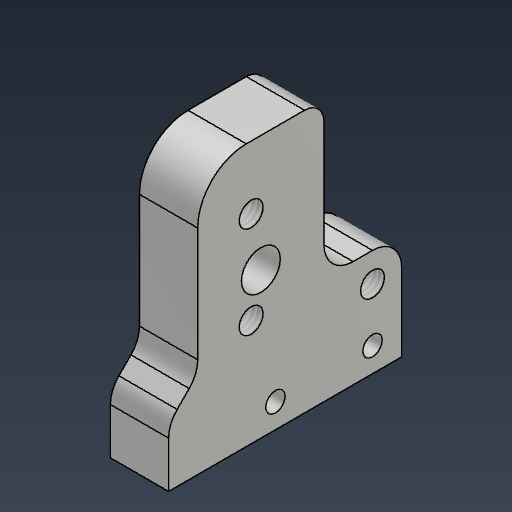
# Autodesk Inventor part: Dribbler Lagerbock v2
Saved by Autodesk Inventor 2023.1 (Build 271208000, 208)
## iProperties
Part Number: Dribbler Lagerbock v2
Material: Aluminium 6061
Document SubType Name: Modeling
Designer: rYan
Mass: 5.82991 g
Surface Area: 16.945 cm^2
Volume: 2.15922 cm^3
Density: 2.7 g/cm^3
Appearance: Aluminium - flach
Author: rYan
Autodesk Inventor part; units mm, degrees
ref_plane "YZ Plane" through (0, 0, 0) normal (1, 0, 0) x (0, 1, 0)
ref_plane "XZ Plane" through (0, 0, 0) normal (0, 1, 0) x (-1, 0, 0)
ref_plane "XY Plane" through (0, 0, 0) normal (0, 0, 1) x (1, 0, 0)
sketch "Skizze1" plane through (0, 0, 0) normal (1, 0, 0) x (0, 1, 0)
  line L0 (6, 0) -> (30, 0)
  line L1 (30, 0) -> (30, 11)
  line L2 (9, 27) -> (9, 9)
  line L3 (9, 27) -> (22, 27)
  line L4 (22, 27) -> (22, 11)
  line L5 (30, 11) -> (22, 11)
  circle A0 centre (15.5, 15) radius 0.5
  circle A1 centre (14.5, 20.5) radius 0.5
  circle A2 centre (27, 8) radius 0.5
  line L6 (0, 32.4) -> (0, -5.4) projected
  line L7 (1.2, 0) -> (34.8, 0) projected
  line L8 (9, 9) -> (6, 6)
  line L9 (6, 6) -> (6, 0)
  circle A3 centre (14.5, 11) radius 0.5
  line L10 (14.5, 20.5) -> (14.5, 11) construction
  dimension "d1" = 11
  dimension "d3" = 27
  dimension "d21" = 1
  dimension "d28" = 1
  dimension "d41" = 1
  dimension "d43" = 8
  dimension "d54" = 9
  dimension "d55" = 27
  dimension "d61" = 15
  dimension "d62" = 15.5
  dimension "d127" = 30
  dimension "d172" = 6
  dimension "d175" = 6
  dimension "d176" = 45
  dimension "d180" = 22
  dimension "d197" = 1
  dimension "d198" = 14.5
  dimension "d199" = 11
  dimension "d201" = 9.5
  dimension "d202" = 0
  constraints: 18 end point, 4 centre point, 2 parallel, 1 collinear, 1 horizontal, 1 perpendicular, 1 point on line, 1 vertical
  measures "d1" distance of L0.end L1.end
  measures "d3" distance between parallel lines of L0 L3
  measures "d21" diameter of A0
  measures "d28" diameter of A1
  measures "d41" diameter of A2
  measures "d43" distance from line of L0 A2.centre
  measures "d54" distance between parallel lines of L6 L2
  measures "d55" distance from line of L6 A2.centre
  measures "d61" distance from line of L0 A0.centre
  measures "d62" distance from line of L6 A0.centre
  measures "d127" distance between parallel lines of L1 L6
  measures "d172" distance of L8.end L0.start
  measures "d175" distance between parallel lines of L9 L6
  measures "d176" angle of L9 L8
  measures "d180" distance between parallel lines of L6 L4
  measures "d197" diameter of A3
  measures "d198" distance from line of L10.end L6
  measures "d199" distance from line of L7 L10.end
  measures "d201" distance of L10.start L10.end
  measures "d202" angle of L6 L10
extrude "Extrusion1" add sketch "Skizze1" along normal mid plane 6
sketch "Skizze9" plane through (-3, 0, 0) normal (-1, 0, 0) x (0, 0, 1)
  circle A0 centre (8, 27) radius 0.5 projected
  point P0 (0, 0)
  constraints: 1 coincident
hole "Feder" at (-3, 27, 8) direction (1, 0, 0) diameter 2.459 end through all thread size "M3x0.5" class "6H" standard "ISO Metric profile"
sketch "Skizze3" plane through (-3, 0, 0) normal (-1, 0, 0) x (0, 0, 1)
  circle A0 centre (20.5, 14.5) radius 0.5 projected
  circle A1 centre (11, 14.5) radius 0.5 projected
  constraints: 2 coincident
hole "Dribbler" at (-3, 14.5, 20.5) at (-3, 14.5, 11) direction (1, 0, 0) diameter 2.459 end through all thread size "M3x0.5" class "6H" standard "ISO Metric profile"
sketch "Skizze4" plane through (-3, 0, 0) normal (-1, 0, 0) x (0, 0, 1)
  circle A0 centre (15, 15.5) radius 0.5 projected
  circle A1 centre (15, 15.5) radius 0.5 projected
  point P0 (0, 0)
  constraints: 1 coincident
hole "Chipper" at (-3, 15.5, 15) direction (1, 0, 0) diameter 4 end through all
sketch "Skizze5" plane through (3, 30, 0) normal (0, 0, -1) x (-1, 0, 0)
  line L0 (6, 0) -> (0, 0) projected
  line L1 (0, -24) -> (0, 0) projected
  line L2 (6, 0) -> (6, -24) projected
  line L3 (3, -24) -> (3, 0) construction
  line L4 (6, -24) -> (0, -24) projected
  line L5 (-1.2, -30) -> (7.2, -30) projected
  point P0 (3, -20.5)
  point P1 (3, -6.5)
  point P2 (3, -13.5)
  point P3 (3, -12)
  dimension "d58" = 7
  dimension "d89" = 7
  dimension "d185" = 9.5
  constraints: 3 midpoint, 3 point on line, 2 end point
  measures "d58" distance of point (3, -13.5) point (3, -20.5)
  measures "d89" distance of point (3, -13.5) point (3, -6.5)
  measures "d185" distance from line of L5 point (3, -20.5)
hole "Montage" at (0, 9.5, 0) at (0, 23.5, 0) direction (0, 0, 1) diameter 2.459 depth 7 tip angle 118 thread size "M3x0.5" class "6H" standard "ISO Metric profile"
fillet "Rundung2" radius 3 4 edges at (0, 22, 11) (0, 30, 11) (0, 9, 9) (0, 6, 6)
sketch "Skizze16" plane through (-3, 0, 0) normal (-1, 0, 0) x (0, 0, 1)
  line L0 (2.5, 27) -> (2.5, 17) construction
  line L1 (0, 36) -> (0, -6) construction
  point P0 (0, 0)
  dimension "d161" = 17
  dimension "d162" = 10
  dimension "d177" = 2.5
  constraints: 2 end point, 1 vertical
  measures "d161" vertical distance of point (0, 0) L0.end
  measures "d162" distance of L0.start L0.end
  measures "d177" horizontal distance of point (0, 0) L0.end
hole "Bohrung10" at (-3, 27, 2.5) at (-3, 17, 2.5) direction (1, 0, 0) diameter 2 end through all
fillet "Rundung7" radius 5 1 edges at (0, 9, 27)
fillet "Rundung8" radius 2 1 edges at (0, 22, 27)
